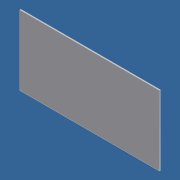
# Autodesk Inventor part: GE-11041-04
Saved by Autodesk Inventor 2012 (Build 160160000, 160)
## iProperties
Created: 2010-10-06
Part Number: GE-11041-04
Document SubType Name: Modeling
Designer: mcyr
Density: 1 g/cm^3
Description: Foot Plate
Material: Default
Title: Foot Plate
Author: mcyr
Autodesk Inventor part; units mm, degrees
ref_plane "YZ Plane" through (0, 0, 0) normal (1, 0, 0) x (0, 1, 0)
ref_plane "XZ Plane" through (0, 0, 0) normal (0, 1, 0) x (-1, 0, 0)
ref_plane "XY Plane" through (0, 0, 0) normal (0, 0, 1) x (1, 0, 0)
sketch "Sketch1" plane through (0, 0, 0) normal (0, 0, 1) x (1, 0, 0)
  line L0 (-25.5063, 25.3616) -> (380.8937, 25.3616)
  line L1 (380.8937, 25.3616) -> (380.8937, -177.8384)
  line L2 (380.8937, -177.8384) -> (-25.5063, -177.8384)
  line L3 (-25.5063, -177.8384) -> (-25.5063, 25.3616)
  point P0 (0, 0)
  dimension "d0" = 406.4
  dimension "d1" = 203.2
  constraints: 8 end point, 2 parallel, 1 horizontal, 1 perpendicular
  measures "d0" distance of L0.start L0.end
  measures "d1" distance of L2.end L0.start
extrude "Extrusion1" add sketch "Sketch1" along normal blind 3.175
body "Solid1"
